Autodesk Fusion 360 part; units mm, degrees
(part 2 of 2)
  line L878 (-48.8114, -148.3999) -> (-48.8431, -148.4136)
  line L879 (-43.0004, -145.5999) -> (-42.9905, -145.5999)
  line L880 (-36.8003, -145.5886) -> (-36.8155, -145.5568)
  line L881 (-30.959, -145.5847) -> (-30.9633, -145.5625)
  line L882 (-48.8004, -145.5999) -> (-48.8004, -145.5886)
  line L883 (-36.8003, -148.4094) -> (-36.8003, -148.3999)
  line L884 (-48.8004, -148.3999) -> (-48.8114, -148.3999)
  line L885 (-36.8003, -148.3999) -> (-36.8116, -148.3999)
  line L886 (-30.9633, -145.5625) -> (-30.9866, -145.5568)
  line L887 (-42.9591, -148.4136) -> (-42.9905, -148.3999)
  line L888 (-24.812, -148.3999) -> (-24.843, -148.4136)
  line L889 (-36.8116, -148.3999) -> (-36.8434, -148.4136)
  line L890 (-36.8377, -148.4373) -> (-36.8155, -148.4411)
  line L891 (-42.9867, -148.4411) -> (-42.963, -148.4373)
  line L892 (-24.812, -145.5999) -> (-24.801, -145.5999)
  line L893 (-36.8155, -148.4411) -> (-36.8003, -148.4094)
  line L894 (-48.8004, -148.4094) -> (-48.8004, -148.3999)
  line L895 (-24.801, -145.5999) -> (-19, -145.5999)
  line L896 (-36.8434, -148.4136) -> (-36.8377, -148.4373)
  line L897 (-36.8003, -148.3999) -> (-36.8003, -145.5999)
  line L898 (-48.8004, -145.5999) -> (-43.0004, -145.5999)
  line L899 (-48.8431, -145.5847) -> (-48.8114, -145.5999)
  line L900 (-24.801, -148.3999) -> (-24.801, -145.5999)
  line L901 (-48.8114, -145.5999) -> (-48.8004, -145.5999)
  line L902 (-42.9905, -148.3999) -> (-43.0004, -148.3999)
  line L903 (-48.8004, -145.5886) -> (-48.8156, -145.5568)
  line L904 (-43.0004, -148.3999) -> (-43.0004, -148.4094)
  line L905 (-42.963, -148.4373) -> (-42.9591, -148.4136)
  line L906 (-42.9591, -145.5847) -> (-42.963, -145.5625)
  line L907 (-24.801, -148.4094) -> (-24.801, -148.3999)
  line L908 (-31.0003, -148.4094) -> (-30.9866, -148.4411)
  line L909 (-24.843, -148.4136) -> (-24.838, -148.4373)
  line L910 (-24.801, -145.5999) -> (-24.801, -145.5886)
  line L911 (-33.8998, -148.3999) -> (-36.8003, -148.3999)
  line L912 (-42.9867, -145.5568) -> (-43.0004, -145.5886)
  line L913 (-43.0004, -145.5999) -> (-43.0004, -148.3999)
  line L914 (-57.544, -159.1843) -> (-57.5123, -159.1995)
  line L915 (-24.838, -148.4373) -> (-24.816, -148.4411)
  line L916 (-21.9, -148.3999) -> (-24.801, -148.3999)
  line L917 (-36.8377, -145.5625) -> (-36.8434, -145.5847)
  line L918 (-24.801, -145.5886) -> (-24.816, -145.5568)
  line L919 (-94.5377, -195.1374) -> (-94.5155, -195.1416)
  line L920 (-94.5003, -192.289) -> (-94.5155, -192.2573)
  line L921 (-36.8003, -145.5999) -> (-31.0003, -145.5999)
  line L922 (-106.5003, -192.3001) -> (-100.7001, -192.3001)
  line L923 (-106.5113, -195.1002) -> (-106.543, -195.114)
  line L924 (-94.5003, -195.1002) -> (-94.5003, -192.3001)
  line L925 (-31.0003, -145.5999) -> (-30.9908, -145.5999)
  line L926 (-100.7001, -192.289) -> (-100.7001, -192.3001)
  line L927 (-100.6905, -195.1002) -> (-100.7001, -195.1002)
  line L928 (-100.7001, -195.1002) -> (-103.5996, -195.1002)
  line L929 (-100.7001, -192.3001) -> (-100.6905, -192.3001)
  line L930 (-119.5999, -200.0005) -> (-119.5999, -209.9996)
  line L931 (-106.5155, -195.1416) -> (-106.5003, -195.1099)
  line L932 (-100.6629, -195.1374) -> (-100.6588, -195.114)
  line L933 (-36.8116, -145.5999) -> (-36.8003, -145.5999)
  line L934 (-94.5113, -195.1002) -> (-94.543, -195.114)
  line L935 (-94.5003, -195.1099) -> (-94.5003, -195.1002)
  line L936 (-106.543, -192.2849) -> (-106.5113, -192.3001)
  line L937 (-106.5003, -195.1002) -> (-106.5003, -192.3001)
  line L938 (-106.5375, -195.1374) -> (-106.5155, -195.1416)
  line L939 (-100.6588, -195.114) -> (-100.6905, -195.1002)
  line L940 (-94.5003, -192.3001) -> (-94.5003, -192.289)
  line L941 (-100.7001, -195.1002) -> (-100.7001, -195.1099)
  line L942 (-119.5999, -209.9996) -> (-19.6, -209.9996)
  line L943 (-94.5113, -192.3001) -> (-94.5003, -192.3001)
  line L944 (-103.5996, -195.1002) -> (-106.5003, -195.1002)
  line L945 (-94.5155, -192.2573) -> (-94.5377, -192.2615)
  line L946 (-94.5003, -195.1002) -> (-94.5113, -195.1002)
  line L947 (-88.7003, -192.3001) -> (-88.6904, -192.3001)
  line L948 (-88.6904, -192.3001) -> (-88.6587, -192.2849)
  line L949 (-106.5003, -192.289) -> (-106.5155, -192.2573)
  line L950 (-94.5377, -192.2615) -> (-94.543, -192.2849)
  line L951 (-88.6587, -192.2849) -> (-88.6629, -192.2615)
  line L952 (-100.6905, -192.3001) -> (-100.6588, -192.2849)
  line L953 (-106.543, -195.114) -> (-106.5375, -195.1374)
  line L954 (-82.5154, -195.1416) -> (-82.5002, -195.1099)
  line L955 (-76.6865, -192.2573) -> (-76.7002, -192.289)
  line L956 (-63.6005, -198.3) -> (-63.5839, -198.3)
  line L957 (-106.5003, -192.3001) -> (-106.5003, -192.289)
  line L958 (-76.7002, -192.3001) -> (-76.7002, -195.1002)
  line L959 (-36.8434, -145.5847) -> (-36.8116, -145.5999)
  line L960 (-19.6, -200.0005) -> (-119.5999, -200.0005)
  line L961 (-100.7001, -192.3001) -> (-100.7001, -195.1002)
  line L962 (-94.543, -195.114) -> (-94.5377, -195.1374)
  line L963 (-94.5155, -195.1416) -> (-94.5003, -195.1099)
  line L964 (-106.5113, -192.3001) -> (-106.5003, -192.3001)
  line L965 (-24.838, -145.5625) -> (-24.843, -145.5847)
  line L966 (-100.7001, -195.1099) -> (-100.6864, -195.1416)
  line L967 (-106.5375, -192.2615) -> (-106.543, -192.2849)
  line L968 (-91.5994, -195.1002) -> (-94.5003, -195.1002)
  line L969 (-100.6864, -195.1416) -> (-100.6629, -195.1374)
  line L970 (-94.543, -192.2849) -> (-94.5113, -192.3001)
  line L971 (-94.5003, -192.3001) -> (-88.7003, -192.3001)
  line L972 (-106.5003, -195.1099) -> (-106.5003, -195.1002)
  line L973 (-76.6907, -192.3001) -> (-76.6589, -192.2849)
  line L974 (-100.6588, -192.2849) -> (-100.6629, -192.2615)
  line L975 (-24.816, -145.5568) -> (-24.838, -145.5625)
  line L976 (-106.5003, -195.1002) -> (-106.5113, -195.1002)
  line L977 (-100.6629, -192.2615) -> (-100.6864, -192.2573)
  line L978 (-106.5155, -192.2573) -> (-106.5375, -192.2615)
  line L979 (-100.6864, -192.2573) -> (-100.7001, -192.289)
  line L980 (-19.6, -209.9996) -> (-19.6, -200.0005)
  line L981 (-82.5002, -195.1099) -> (-82.5002, -195.1002)
  line L982 (-88.7003, -195.1002) -> (-91.5994, -195.1002)
  line L983 (-88.6629, -192.2615) -> (-88.6865, -192.2573)
  line L984 (-63.5, -198.1994) -> (-63.5, -189.1995)
  line L985 (-76.7002, -192.289) -> (-76.7002, -192.3001)
  line L986 (-63.5839, -189.1003) -> (-63.6005, -189.1003)
  line L987 (-63.6005, -189.1003) -> (-66.5, -189.1003)
  line L988 (-82.5376, -192.2615) -> (-82.5433, -192.2849)
  line L989 (-58.9992, -136.4097) -> (-58.9855, -136.4414)
  line L990 (-58.958, -124.4138) -> (-58.9897, -124.4)
  line L991 (-58.958, -136.4135) -> (-58.9897, -136.3998)
  line L992 (-17.416, -114.752) -> (-17.607, -114.989)
  line L993 (-58.9855, -136.4414) -> (-58.9622, -136.4372)
  line L994 (-58.9897, -124.4) -> (-58.9992, -124.4)
  line L995 (-61.9181, -124.4) -> (-61.9703, -124.429)
  line L996 (-18.597, -115.4) -> (-58.9001, -115.4)
  line L997 (-17.844, -115.181) -> (-17.897, -115.213)
  line L998 (-61.9181, -136.3998) -> (-61.9703, -136.4287)
  line L999 (-61.9993, -130.5006) -> (-61.9993, -130.5172)
  line L1000 (-58.9992, -130.5998) -> (-58.9992, -136.3998)
  line L1001 (-17.353, -114.646) -> (-17.384, -114.7)
  line L1002 (-17.148, -113.254) -> (-17.196, -113.812)
  line L1003 (-58.9622, -124.4371) -> (-58.958, -124.4138)
  line L1004 (-58.9622, -136.4372) -> (-58.958, -136.4135)
  line L1005 (-58.9992, -115.501) -> (-58.9992, -124.4)
  line L1006 (-58.9855, -130.5571) -> (-58.9992, -130.5888)
  line L1007 (-58.9622, -130.5627) -> (-58.9855, -130.5571)
  line L1008 (-17.95, -115.243) -> (-18.234, -115.352)
  line L1009 (-17.196, -114.089) -> (-17.245, -114.362)
  line L1010 (-58.9992, -142.5999) -> (-58.9897, -142.5999)
  line L1011 (-58.9992, -124.4) -> (-61.9001, -124.4)
  line L1012 (-61.9703, -130.5708) -> (-61.9181, -130.5998)
  line L1013 (-17.004, -112.524) -> (-17.148, -113.254)
  line L1014 (-58.9001, -115.4) -> (-58.9181, -115.4)
  line L1015 (-58.9181, -115.4) -> (-58.9703, -115.429)
  line L1016 (-58.9703, -115.429) -> (-58.9992, -115.483)
  line L1017 (-61.9001, -136.3998) -> (-61.9181, -136.3998)
  line L1018 (-12.735, -112.462) -> (-12.74, -112.485)
  line L1019 (-58.9992, -136.3998) -> (-58.9992, -136.4097)
  line L1020 (-61.9993, -124.5006) -> (-61.9993, -130.5006)
  line L1021 (-58.9992, -151.517) -> (-58.9703, -151.5706)
  line L1022 (-10.299, -115.301) -> (-12.697, -115.301)
  line L1023 (-58.958, -130.5846) -> (-58.9622, -130.5627)
  line L1024 (-18.234, -115.352) -> (-18.507, -115.4)
  line L1025 (-61.9001, -124.4) -> (-61.9181, -124.4)
  line L1026 (-61.9703, -142.5709) -> (-61.9181, -142.5999)
  line L1027 (-61.9993, -124.4826) -> (-61.9993, -124.5006)
  line L1028 (-10.29, -115.301) -> (-10.299, -115.301)
  line L1029 (-10.258, -115.315) -> (-10.29, -115.301)
  line L1030 (-10.286, -112.458) -> (-10.299, -112.49)
  line L1031 (-58.9992, -130.5998) -> (-58.9897, -130.5998)
  line L1032 (-18.507, -115.4) -> (-18.597, -115.4)
  line L1033 (-10.286, -115.342) -> (-10.262, -115.338)
  line L1034 (-12.708, -115.301) -> (-12.74, -115.315)
  line L1035 (-12.697, -112.5) -> (-11.498, -112.5)
  line L1036 (-12.735, -115.338) -> (-12.712, -115.342)
  line L1037 (-61.9181, -130.5998) -> (-61.9001, -130.5998)
  line L1038 (-12.697, -115.301) -> (-12.697, -112.5)
  line L1039 (-17.607, -114.989) -> (-17.844, -115.181)
  line L1040 (-58.9897, -130.5998) -> (-58.958, -130.5846)
  line L1041 (-58.9897, -142.5999) -> (-58.958, -142.5847)
  line L1042 (-61.9703, -124.429) -> (-61.9993, -124.4826)
  line L1043 (-17.384, -114.7) -> (-17.416, -114.752)
  line L1044 (-61.9993, -142.5169) -> (-61.9703, -142.5709)
  line L1045 (-58.9992, -124.4) -> (-58.9992, -124.4096)
  line L1046 (-58.9622, -142.5625) -> (-58.9855, -142.5572)
  line L1047 (-61.9001, -130.5998) -> (-58.9992, -130.5998)
  line L1048 (-17.196, -113.812) -> (-17.196, -114)
  line L1049 (-58.9992, -115.483) -> (-58.9992, -115.501)
  line L1050 (-58.9855, -124.4413) -> (-58.9622, -124.4371)
  line L1051 (-17.897, -115.213) -> (-17.95, -115.243)
  line L1052 (-58.9992, -124.4096) -> (-58.9855, -124.4413)
  line L1053 (-10.299, -112.5) -> (-10.29, -112.5)
  line L1054 (-58.9992, -142.5886) -> (-58.9992, -142.5999)
  line L1055 (-12.697, -115.31) -> (-12.697, -115.301)
  line L1056 (-12.74, -112.485) -> (-12.708, -112.5)
  line L1057 (-10.258, -112.485) -> (-10.262, -112.462)
  line L1058 (-10.262, -112.462) -> (-10.286, -112.458)
  line L1059 (-18.991, -145.5999) -> (-18.959, -145.5847)
  line L1060 (-10.299, -112.5) -> (-10.299, -115.301)
  line L1061 (-12.712, -115.342) -> (-12.697, -115.31)
  line L1062 (-58.9181, -151.5996) -> (-58.9001, -151.5996)
  line L1063 (-18.959, -145.5847) -> (-18.963, -145.5625)
  line L1064 (-58.9992, -142.5999) -> (-58.9992, -151.5004)
  line L1065 (-10.299, -115.31) -> (-10.286, -115.342)
  line L1066 (-58.9703, -151.5706) -> (-58.9181, -151.5996)
  line L1067 (-10.262, -115.338) -> (-10.258, -115.315)
  line L1068 (-11.498, -112.5) -> (-10.299, -112.5)
  line L1069 (-12.697, -112.5) -> (-12.697, -112.49)
  line L1070 (-10.29, -112.5) -> (-10.258, -112.485)
  line L1071 (-58.9855, -142.5572) -> (-58.9992, -142.5886)
  line L1072 (-58.9992, -151.5004) -> (-58.9992, -151.517)
  line L1073 (-58.958, -142.5847) -> (-58.9622, -142.5625)
  line L1074 (-10.299, -112.49) -> (-10.299, -112.5)
  line L1075 (-12.697, -112.49) -> (-12.712, -112.458)
  line L1076 (-12.697, -115.301) -> (-12.708, -115.301)
  line L1077 (-12.74, -115.315) -> (-12.735, -115.338)
  line L1078 (-10.299, -115.301) -> (-10.299, -115.31)
  line L1079 (-12.708, -112.5) -> (-12.697, -112.5)
  line L1080 (-12.712, -112.458) -> (-12.735, -112.462)
  line L1081 (-19, -145.5999) -> (-18.991, -145.5999)
  line L1082 (-8.829, -115.429) -> (-8.883, -115.4)
  line L1083 (-10.077, -116.53) -> (-10.168, -116.578)
  line L1084 (-13.862, -115.681) -> (-14.075, -115.328)
  line L1085 (-10.261, -116.625) -> (-10.55, -116.739)
  line L1086 (-8.837, -124.4371) -> (-8.815, -124.4413)
  line L1087 (-14.341, -113.416) -> (-14.316, -113.316)
  line L1088 (-8.883, -115.4) -> (-8.899, -115.4)
  line L1089 (-14.238, -114.948) -> (-14.272, -114.85)
  line L1090 (-8.899, -115.4) -> (-8.921, -115.4)
  line L1091 (-11.672, -116.896) -> (-11.774, -116.887)
  line L1092 (-61.9993, -130.5172) -> (-61.9703, -130.5708)
  line L1093 (-17.196, -114) -> (-17.196, -114.089)
  line L1094 (-9, -115.513) -> (-8.989, -115.546)
  line L1095 (-9.077, -112.401) -> (-8.921, -112.672)
  line L1096 (-8.649, -109.065) -> (-8.811, -108.971)
  line L1097 (-13.575, -111.971) -> (-13.499, -111.901)
  line L1098 (-5.8, -115.517) -> (-5.8, -115.501)
  line L1099 (-16.018, -110.53) -> (-16.341, -110.99)
  line L1100 (-9.137, -112.317) -> (-9.077, -112.401)
  line L1101 (-8.921, -112.672) -> (-8.759, -113.05)
  line L1102 (-5.829, -115.571) -> (-5.8, -115.517)
  line L1103 (-8.912, -115.6) -> (-8.899, -115.6)
  line L1104 (-8.811, -108.971) -> (-9.32, -108.735)
  line L1105 (-8.759, -113.05) -> (-8.651, -113.45)
  line L1106 (-16.764, -111.82) -> (-17.004, -112.524)
  line L1107 (-53.5284, -161.5504) -> (-53.5615, -161.6484)
  line L1108 (-58.3036, -162.7978) -> (-58.5819, -162.493)
  line L1109 (-58.958, -171.1142) -> (-58.9897, -171.1004)
  line L1110 (-55.1021, -161.9998) -> (-55.1021, -162.0093)
  line L1111 (-61.9181, -177.3001) -> (-61.9001, -177.3001)
  line L1112 (-61.9001, -171.1004) -> (-61.9181, -171.1004)
  line L1113 (-58.7622, -162.2383) -> (-58.8133, -162.1501)
  line L1114 (-57.9864, -163.061) -> (-58.3036, -162.7978)
  line L1115 (-58.9992, -162.1995) -> (-58.9992, -171.1004)
  line L1116 (-58.958, -177.285) -> (-58.9622, -177.2617)
  line L1117 (-53.9404, -162.3815) -> (-54.2039, -162.6997)
  line L1118 (-58.9992, -183.1002) -> (-58.9992, -183.11)
  line L1119 (-57.5402, -163.3241) -> (-57.6308, -163.2772)
  line L1120 (-61.9703, -177.2698) -> (-61.9181, -177.3001)
  line L1121 (-58.8133, -162.1501) -> (-58.819, -162.1416)
  line L1122 (-58.819, -162.1416) -> (-58.8807, -162.1003)
  line L1123 (-56.8508, -163.5474) -> (-57.2505, -163.4398)
  line L1124 (-55.9248, -163.5764) -> (-56.0267, -163.5873)
  line L1125 (-53.4596, -160.116) -> (-53.4155, -160.4247)
  line L1126 (-58.5819, -162.493) -> (-58.7622, -162.2383)
  line L1127 (-58.8807, -162.1003) -> (-58.9001, -162.1003)
  line L1128 (-58.9897, -177.3001) -> (-58.958, -177.285)
  line L1129 (-58.9622, -171.1375) -> (-58.958, -171.1142)
  line L1130 (-55.6175, -163.5171) -> (-55.9248, -163.5764)
  line L1131 (-58.9001, -162.1003) -> (-58.9181, -162.1003)
  line L1132 (-56.1301, -163.5968) -> (-56.4416, -163.5954)
  line L1133 (-53.4553, -161.2473) -> (-53.5284, -161.5504)
  line L1134 (-58.9855, -171.1417) -> (-58.9622, -171.1375)
  line L1135 (-58.9992, -171.1004) -> (-61.9001, -171.1004)
  line L1136 (-58.9992, -171.1099) -> (-58.9855, -171.1417)
  line L1137 (-53.5079, -159.9163) -> (-53.4832, -160.0168)
  line L1138 (-5.8, -114) -> (-5.8, -113.812)
  line L1139 (-12.244, -108.35) -> (-12.974, -108.495)
  line L1140 (-9, -115.488) -> (-9, -115.501)
  line L1141 (-8.986, -115.45) -> (-8.989, -115.453)
  line L1142 (-10.754, -108.35) -> (-11.312, -108.302)
  line L1143 (-11.312, -108.302) -> (-11.498, -108.302)
  line L1144 (-11.498, -108.302) -> (-11.686, -108.302)
  line L1145 (-8.651, -113.45) -> (-8.607, -113.759)
  line L1146 (-14.187, -108.971) -> (-14.347, -109.065)
  line L1147 (-8.955, -115.583) -> (-8.95, -115.586)
  line L1148 (-8.598, -113.964) -> (-8.613, -114.276)
  line L1149 (-14.968, -109.48) -> (-15.528, -109.97)
  line L1150 (-14.347, -109.065) -> (-14.508, -109.158)
  line L1151 (-13.679, -108.735) -> (-14.187, -108.971)
  line L1152 (-61.9703, -171.1293) -> (-61.9993, -171.1816)
  line L1153 (-53.5615, -161.6484) -> (-53.5961, -161.7447)
  line L1154 (-57.6308, -163.2772) -> (-57.7232, -163.2289)
  line L1155 (-61.9993, -171.1995) -> (-61.9993, -177.1996)
  line L1156 (-58.9855, -177.2574) -> (-58.9992, -177.2892)
  line L1157 (-58.9992, -177.2892) -> (-58.9992, -177.3001)
  line L1158 (-58.9897, -171.1004) -> (-58.9992, -171.1004)
  line L1159 (-58.9992, -177.3001) -> (-58.9992, -183.1002)
  line L1160 (-61.9993, -171.1816) -> (-61.9993, -171.1995)
  line L1161 (-61.9993, -177.2162) -> (-61.9703, -177.2698)
  line L1162 (-54.8541, -163.2109) -> (-55.2249, -163.3915)
  line L1163 (-56.4416, -163.5954) -> (-56.8508, -163.5474)
  line L1164 (-57.2505, -163.4398) -> (-57.5402, -163.3241)
  line L1165 (-53.4832, -160.0168) -> (-53.4596, -160.116)
  line L1166 (-58.9181, -162.1003) -> (-58.9703, -162.1293)
  line L1167 (-61.9993, -136.4827) -> (-61.9993, -136.5007)
  line L1168 (-61.9993, -136.5007) -> (-61.9993, -142.5004)
  line L1169 (-58.9992, -136.3998) -> (-61.9001, -136.3998)
  line L1170 (-58.9992, -130.5888) -> (-58.9992, -130.5998)
  line L1171 (-76.5157, -69.741) -> (-76.5005, -69.71)
  line L1172 (-82.6629, -69.737) -> (-82.659, -69.714)
  line L1173 (-94.6905, -69.7) -> (-94.7, -69.7)
  line L1174 (-94.7, -69.7) -> (-100.5003, -69.7)
  line L1175 (-63.6005, -79.701) -> (-66.5, -79.701)
  line L1176 (-63.5839, -79.701) -> (-63.6005, -79.701)
  line L1177 (-94.6174, -66.7) -> (-94.6711, -66.729)
  line L1178 (-94.7, -69.7) -> (-94.7, -69.71)
  line L1179 (-66.5152, -79.742) -> (-66.5, -79.71)
  line L1180 (-82.7003, -66.799) -> (-82.7003, -69.7)
  line L1181 (-66.5, -79.701) -> (-66.5, -69.799)
  line L1182 (-88.5377, -69.737) -> (-88.5154, -69.741)
  line L1183 (-63.5, -79.782) -> (-63.5303, -79.73)
  line L1184 (-76.5005, -69.7) -> (-76.5005, -66.799)
  line L1185 (-82.6174, -66.7) -> (-82.6713, -66.729)
  line L1186 (-66.5825, -69.7) -> (-66.5991, -69.7)
  line L1187 (-76.5115, -69.7) -> (-76.5432, -69.714)
  line L1188 (-82.6907, -69.7) -> (-82.7003, -69.7)
  line L1189 (-100.5155, -69.741) -> (-100.5003, -69.71)
  line L1190 (-116.7006, -91.71) -> (-116.6868, -91.742)
  line L1191 (-76.5376, -69.737) -> (-76.5157, -69.741)
  line L1192 (-82.659, -69.714) -> (-82.6907, -69.7)
  line L1193 (-88.5003, -69.7) -> (-88.5116, -69.7)
  line L1194 (-82.5997, -66.7) -> (-82.6174, -66.7)
  line L1195 (-94.7, -69.71) -> (-94.6862, -69.741)
  line L1196 (-94.6711, -66.729) -> (-94.7, -66.782)
  line L1197 (-76.5005, -69.7) -> (-76.5115, -69.7)
  line L1198 (-66.5, -79.71) -> (-66.5, -79.701)
  line L1199 (-94.663, -69.737) -> (-94.6587, -69.714)
  line L1200 (-94.6587, -69.714) -> (-94.6905, -69.7)
  line L1201 (-66.5, -79.701) -> (-66.5109, -79.701)
  line L1202 (-76.5997, -66.7) -> (-82.5997, -66.7)
  line L1203 (-82.7003, -66.782) -> (-82.7003, -66.799)
  line L1204 (-94.6862, -69.741) -> (-94.663, -69.737)
  line L1205 (-8.935, -115.36) -> (-8.986, -115.45)
  line L1206 (-5.994, -112.524) -> (-6.234, -111.82)
  line L1207 (-14.508, -109.158) -> (-14.968, -109.48)
  line L1208 (-61.9703, -136.4287) -> (-61.9993, -136.4827)
  line L1209 (-6.234, -111.82) -> (-6.471, -111.311)
  line L1210 (-6.657, -110.989) -> (-6.98, -110.53)
  line L1211 (-7.47, -109.97) -> (-8.028, -109.48)
  line L1212 (-8.947, -115.587) -> (-8.912, -115.6)
  line L1213 (-5.883, -115.6) -> (-5.829, -115.571)
  line L1214 (-5.85, -113.254) -> (-5.994, -112.524)
  line L1215 (-53.4059, -160.8381) -> (-53.4553, -161.2473)
  line L1216 (-61.9993, -177.1996) -> (-61.9993, -177.2162)
  line L1217 (-54.5098, -162.9795) -> (-54.5909, -163.043)
  line L1218 (-58.9622, -177.2617) -> (-58.9855, -177.2574)
  line L1219 (-58.8807, -159.372) -> (-58.7251, -159.1017)
  line L1220 (-61.9181, -162.3) -> (-61.9001, -162.3)
  line L1221 (-58.8161, -162.2535) -> (-58.8133, -162.2506)
  line L1222 (-59.1993, -160.5626) -> (-59.195, -160.4592)
  line L1223 (-61.9509, -159.9548) -> (-61.9993, -160.5128)
  line L1224 (-54.4297, -162.9149) -> (-54.5098, -162.9795)
  line L1225 (-61.9993, -160.7002) -> (-61.9993, -162.1995)
  line L1226 (-61.9181, -171.1004) -> (-61.9703, -171.1293)
  line L1227 (-58.9992, -177.3001) -> (-58.9897, -177.3001)
  line L1228 (-61.9001, -177.3001) -> (-58.9992, -177.3001)
  line L1229 (-54.2039, -162.6997) -> (-54.4297, -162.9149)
  line L1230 (-58.9992, -162.1815) -> (-58.9992, -162.1995)
  line L1231 (-53.4155, -160.4247) -> (-53.4059, -160.8381)
  line L1232 (-53.5961, -161.7447) -> (-53.7256, -162.0287)
  line L1233 (-57.7232, -163.2289) -> (-57.9864, -163.061)
  line L1234 (-54.5909, -163.043) -> (-54.8541, -163.2109)
  line L1235 (-58.9703, -162.1293) -> (-58.9992, -162.1815)
  line L1236 (-53.7256, -162.0287) -> (-53.9404, -162.3815)
  line L1237 (-55.2249, -163.3915) -> (-55.6175, -163.5171)
  line L1238 (-58.9992, -171.1004) -> (-58.9992, -171.1099)
  line L1239 (-56.0267, -163.5873) -> (-56.1301, -163.5968)
  line L1240 (-82.6713, -66.729) -> (-82.7003, -66.782)
  line L1241 (-66.5152, -85.858) -> (-66.537, -85.862)
  line L1242 (-66.5109, -91.7) -> (-66.5427, -91.714)
  line L1243 (-66.5427, -85.885) -> (-66.5109, -85.9)
  line L1244 (-66.5, -103.7) -> (-66.5109, -103.7)
  line L1245 (-66.537, -91.738) -> (-66.5152, -91.742)
  line L1246 (-66.5, -103.7) -> (-66.5, -97.9)
  line L1247 (-63.6005, -97.9) -> (-63.5839, -97.9)
  line L1248 (-63.6005, -85.9) -> (-63.5839, -85.9)
  line L1249 (-66.5, -91.7) -> (-66.5, -85.9)
  line L1250 (-66.5109, -85.9) -> (-66.5, -85.9)
  line L1251 (-63.5839, -91.7) -> (-63.6005, -91.7)
  line L1252 (-63.5839, -85.9) -> (-63.5303, -85.87)
  line L1253 (-66.537, -85.862) -> (-66.5427, -85.885)
  line L1254 (-66.5, -119.817) -> (-66.5, -119.8)
  line L1255 (-66.5427, -91.714) -> (-66.537, -91.738)
  line L1256 (-66.5152, -103.742) -> (-66.5, -103.71)
  line L1257 (-66.537, -97.862) -> (-66.5427, -97.885)
  line L1258 (-66.5109, -109.9) -> (-66.5, -109.9)
  line L1259 (-63.5303, -85.87) -> (-63.5, -85.816)
  line L1260 (-66.5109, -97.9) -> (-66.5, -97.9)
  line L1261 (-63.5839, -103.7) -> (-63.6005, -103.7)
  line L1262 (-63.5, -109.816) -> (-63.5, -109.8)
  line L1263 (-66.5, -109.9) -> (-66.5, -109.889)
  line L1264 (-66.5, -97.9) -> (-66.5, -97.889)
  line L1265 (-63.5, -97.8) -> (-63.5, -91.8)
  line L1266 (-66.537, -109.862) -> (-66.5427, -109.885)
  line L1267 (-66.5, -109.9) -> (-63.6005, -109.9)
  line L1268 (-63.5, -91.782) -> (-63.5303, -91.729)
  line L1269 (-66.5303, -69.729) -> (-66.5825, -69.7)
  line L1270 (-55.3529, -157.9594) -> (-54.9726, -158.1221)
  line L1271 (-54.9726, -158.1221) -> (-54.6213, -158.3369)
  line L1272 (-59.1206, -161.3839) -> (-59.1894, -160.9757)
  line L1273 (-56.5781, -157.812) -> (-56.1661, -157.8021)
  line L1274 (-58.6645, -159.0178) -> (-58.6052, -158.9335)
  line L1275 (-59.1495, -160.1505) -> (-59.0433, -159.7508)
  line L1276 (-59.2046, -160.6645) -> (-59.1993, -160.5626)
  line L1277 (-55.8546, -157.8324) -> (-55.7526, -157.8533)
  line L1278 (-61.8063, -159.2245) -> (-61.9509, -159.9548)
  line L1279 (-59.1894, -160.9757) -> (-59.2046, -160.6645)
  line L1280 (-56.1661, -157.8021) -> (-55.8546, -157.8324)
  line L1281 (-58.8655, -162.0605) -> (-58.9954, -161.7765)
  line L1282 (-55.7526, -157.8533) -> (-55.6521, -157.8727)
  line L1283 (-58.6052, -158.9335) -> (-58.4013, -158.6967)
  line L1284 (-59.195, -160.4592) -> (-59.1495, -160.1505)
  line L1285 (-58.0954, -158.4195) -> (-57.7536, -158.188)
  line L1286 (-61.5668, -158.5204) -> (-61.8063, -159.2245)
  line L1287 (-58.7996, -162.1995) -> (-58.7996, -162.1871)
  line L1288 (-58.7996, -162.1871) -> (-58.8119, -162.1526)
  line L1289 (-58.8546, -162.2877) -> (-58.8504, -162.2863)
  line L1290 (-58.8479, -162.2838) -> (-58.8161, -162.2535)
  line L1291 (-58.8504, -162.2863) -> (-58.8479, -162.2838)
  line L1292 (-58.9001, -162.3) -> (-58.8878, -162.3)
  line L1293 (-61.9703, -162.2697) -> (-61.9181, -162.3)
  line L1294 (-61.3297, -158.0117) -> (-61.5668, -158.5204)
  line L1295 (-57.38, -158.0074) -> (-57.2851, -157.969)
  line L1296 (-56.9859, -157.8808) -> (-56.5781, -157.812)
  line L1297 (-55.6521, -157.8727) -> (-55.3529, -157.9594)
  line L1298 (-61.1434, -157.6892) -> (-61.2359, -157.8504)
  line L1299 (-58.8119, -162.2464) -> (-58.7996, -162.2104)
  line L1300 (-57.2851, -157.969) -> (-56.9859, -157.8808)
  line L1301 (-59.7725, -156.1804) -> (-60.3306, -156.6707)
  line L1302 (-58.8878, -162.3) -> (-58.8546, -162.2877)
  line L1303 (-58.4013, -158.6967) -> (-58.0954, -158.4195)
  line L1304 (-58.8133, -162.1501) -> (-58.8655, -162.0605)
  line L1305 (-61.9993, -162.1995) -> (-61.9993, -162.2161)
  line L1306 (-58.8119, -162.1526) -> (-58.8133, -162.1501)
  line L1307 (-50.6042, -160.5128) -> (-50.6539, -159.9548)
  line L1308 (-51.4614, -157.6892) -> (-51.7839, -157.2288)
  line L1309 (-8.815, -177.2574) -> (-8.837, -177.2617)
  line L1310 (-5.8, -171.1995) -> (-5.8, -171.1816)
  line L1311 (-8.8, -162.1815) -> (-8.829, -162.1293)
  line L1312 (-8.8, -171.1004) -> (-8.8, -162.1995)
  line L1313 (-53.6155, -155.6717) -> (-54.1238, -155.4346)
  line L1314 (-55.5582, -155.0504) -> (-56.1163, -155.0021)
  line L1315 (-8.815, -171.1417) -> (-8.8, -171.1099)
  line L1316 (-8.8, -177.3001) -> (-5.899, -177.3001)
  line L1317 (-8.843, -171.1142) -> (-8.837, -171.1375)
  line L1318 (-8.811, -177.3001) -> (-8.8, -177.3001)
  line L1319 (-8.8, -171.1099) -> (-8.8, -171.1004)
  line L1320 (-5.899, -171.1004) -> (-8.8, -171.1004)
  line L1321 (-5.883, -177.3001) -> (-5.829, -177.2698)
  line L1322 (-51.7839, -157.2288) -> (-52.2746, -156.6707)
  line L1323 (-17.245, -114.362) -> (-17.353, -114.646)
  line L1324 (-58.9897, -136.3998) -> (-58.9992, -136.3998)
  line L1325 (-58.8133, -162.2506) -> (-58.8119, -162.2464)
  line L1326 (-60.821, -157.2288) -> (-61.1434, -157.6892)
  line L1327 (-8.811, -171.1004) -> (-8.843, -171.1142)
  line L1328 (-49.9043, -161.913) -> (-49.9579, -161.8813)
  line L1329 (-8.843, -177.285) -> (-8.811, -177.3001)
  line L1330 (-8.8, -171.1004) -> (-8.811, -171.1004)
  line L1331 (-8.8, -162.1995) -> (-8.8, -162.1815)
  line L1332 (-50.6042, -160.7002) -> (-50.6042, -160.5128)
  line L1333 (-50.4155, -161.4004) -> (-50.4472, -161.3465)
  line L1334 (-5.8, -177.1996) -> (-5.8, -171.1995)
  line L1335 (-5.8, -171.1816) -> (-5.829, -171.1293)
  line L1336 (-58.7251, -159.1017) -> (-58.6645, -159.0178)
  line L1337 (-57.4766, -158.0448) -> (-57.38, -158.0074)
  line L1338 (-61.9993, -160.5128) -> (-61.9993, -160.7002)
  line L1339 (-59.3122, -155.8579) -> (-59.7725, -156.1804)
  line L1340 (-6.471, -111.311) -> (-6.564, -111.151)
  line L1341 (-5.8, -115.501) -> (-5.8, -114)
  line L1342 (-15.528, -109.97) -> (-16.018, -110.53)
  line L1343 (-8.607, -113.759) -> (-8.602, -113.862)
  line L1344 (-10.024, -108.495) -> (-10.754, -108.35)
  line L1345 (-119.7005, -79.8) -> (-119.7005, -85.8)
  line L1346 (-116.7006, -79.701) -> (-116.7006, -79.71)
  line L1347 (-106.6588, -69.714) -> (-106.6905, -69.7)
  line L1348 (-116.6592, -85.885) -> (-116.6633, -85.862)
  line L1349 (-119.7005, -85.816) -> (-119.6716, -85.87)
  line L1350 (-116.6868, -85.858) -> (-116.7006, -85.889)
  line L1351 (-116.7006, -85.889) -> (-116.7006, -85.9)
  line L1352 (-116.6633, -85.862) -> (-116.6868, -85.858)
  line L1353 (-119.5999, -85.9) -> (-116.7006, -85.9)
  line L1354 (-119.6716, -103.729) -> (-119.7005, -103.782)
  line L1355 (-116.6592, -109.885) -> (-116.6633, -109.862)
  line L1356 (-116.6633, -109.862) -> (-116.6868, -109.857)
  line L1357 (-116.6179, -69.7) -> (-116.6716, -69.729)
  line L1358 (-100.5293, -66.729) -> (-100.583, -66.7)
  line L1359 (-106.7001, -66.782) -> (-106.7001, -66.799)
  line L1360 (-119.6179, -79.701) -> (-119.6716, -79.73)
  line L1361 (-106.6864, -69.741) -> (-106.6629, -69.737)
  line L1362 (-100.5114, -69.7) -> (-100.5431, -69.714)
  line L1363 (-106.6905, -69.7) -> (-106.7001, -69.7)
  line L1364 (-3.6005, -61.696) -> (-6.5, -61.696)
  line L1365 (-3.5, -61.795) -> (-3.5, -61.777)
  line L1366 (-116.6909, -109.9) -> (-116.6592, -109.885)
  line L1367 (-116.7006, -91.7) -> (-116.7006, -91.71)
  line L1368 (-119.7005, -85.8) -> (-119.7005, -85.816)
  line L1369 (-116.6592, -79.714) -> (-116.6909, -79.701)
  line L1370 (-119.7005, -79.782) -> (-119.7005, -79.8)
  line L1371 (-116.6716, -119.87) -> (-116.6179, -119.901)
  line L1372 (-119.7005, -97.816) -> (-119.6716, -97.87)
  line L1373 (-6.5, -61.696) -> (-6.5109, -61.696)
  line L1374 (-116.7006, -109.889) -> (-116.7006, -109.9)
  line L1375 (-100.5003, -69.71) -> (-100.5003, -69.7)
  line L1376 (-116.6592, -97.885) -> (-116.6633, -97.862)
  line L1377 (-3.5303, -105.17) -> (-3.5, -105.117)
  line L1378 (-119.5999, -79.701) -> (-119.6179, -79.701)
  line L1379 (-116.7006, -69.782) -> (-116.7006, -69.799)
  line L1380 (-3.5839, -61.696) -> (-3.6005, -61.696)
  line L1381 (-116.7006, -79.701) -> (-119.5999, -79.701)
  line L1382 (-119.5999, -109.9) -> (-116.7006, -109.9)
  line L1383 (-119.7005, -97.8) -> (-119.7005, -97.816)
  line L1384 (-116.6179, -119.901) -> (-116.5999, -119.901)
  line L1385 (-6.537, -61.733) -> (-6.5152, -61.737)
  line L1386 (-6.5152, -56.055) -> (-6.537, -56.058)
  line L1387 (-6.5109, -61.696) -> (-6.5427, -61.71)
  line L1388 (-116.6909, -103.7) -> (-116.7006, -103.7)
  line L1389 (-116.6909, -97.9) -> (-116.6592, -97.885)
  line L1390 (-116.7006, -97.9) -> (-116.6909, -97.9)
  line L1391 (-116.6868, -91.742) -> (-116.6633, -91.738)
  line L1392 (-106.7001, -66.799) -> (-106.7001, -69.7)
  line L1393 (-116.6633, -91.738) -> (-116.6592, -91.714)
  line L1394 (-116.6633, -79.738) -> (-116.6592, -79.714)
  line L1395 (-116.6868, -79.742) -> (-116.6633, -79.738)
  line L1396 (-119.6179, -85.9) -> (-119.5999, -85.9)
  line L1397 (-116.7006, -85.9) -> (-116.7006, -91.7)
  line L1398 (-106.6629, -69.737) -> (-106.6588, -69.714)
  line L1399 (-116.6592, -91.714) -> (-116.6909, -91.7)
  line L1400 (-116.6909, -91.7) -> (-116.7006, -91.7)
  line L1401 (-116.7006, -91.7) -> (-119.5999, -91.7)
  line L1402 (-119.5999, -91.7) -> (-119.6179, -91.7)
  line L1403 (-100.5431, -69.714) -> (-100.5376, -69.737)
  line L1404 (-119.6716, -85.87) -> (-119.6179, -85.9)
  line L1405 (-116.7006, -69.799) -> (-116.7006, -79.701)
  line L1406 (-106.7001, -69.7) -> (-116.5999, -69.7)
  line L1407 (-116.5999, -69.7) -> (-116.6179, -69.7)
  line L1408 (-116.6909, -85.9) -> (-116.6592, -85.885)
  line L1409 (-106.7001, -69.71) -> (-106.6864, -69.741)
  line L1410 (-100.5376, -69.737) -> (-100.5155, -69.741)
  line L1411 (-116.6716, -69.729) -> (-116.7006, -69.782)
  line L1412 (-116.6909, -79.701) -> (-116.7006, -79.701)
  line L1413 (-119.6716, -79.73) -> (-119.7005, -79.782)
  line L1414 (-106.6712, -66.729) -> (-106.7001, -66.782)
  line L1415 (-100.583, -66.7) -> (-100.5996, -66.7)
  line L1416 (-100.5003, -69.7) -> (-100.5003, -66.799)
  line L1417 (-106.7001, -69.7) -> (-106.7001, -69.71)
  line L1418 (-106.5995, -66.7) -> (-106.6174, -66.7)
  line L1419 (-100.5003, -66.782) -> (-100.5293, -66.729)
  line L1420 (-116.7006, -79.71) -> (-116.6868, -79.742)
  line L1421 (-116.7006, -85.9) -> (-116.6909, -85.9)
  line L1422 (-119.6716, -91.729) -> (-119.7005, -91.782)
  line L1423 (-100.5996, -66.7) -> (-106.5995, -66.7)
  line L1424 (-100.5003, -66.799) -> (-100.5003, -66.782)
  line L1425 (-100.5003, -69.7) -> (-100.5114, -69.7)
  line L1426 (-106.6174, -66.7) -> (-106.6712, -66.729)
  line L1427 (-119.6179, -91.7) -> (-119.6716, -91.729)
  line L1428 (-119.7005, -91.782) -> (-119.7005, -91.8)
  line L1429 (-19, -195.1002) -> (-21.9, -195.1002)
  line L1430 (-24.801, -192.3001) -> (-24.801, -192.289)
  line L1431 (-18.991, -192.3001) -> (-18.959, -192.2849)
  line L1432 (-8.8, -189.289) -> (-8.815, -189.2574)
  line L1433 (-5.899, -189.3001) -> (-5.883, -189.3001)
  line L1434 (-8.899, -198.3) -> (-8.883, -198.3)
  line L1435 (-18.963, -192.2615) -> (-18.986, -192.2573)
  line L1436 (-24.843, -195.114) -> (-24.838, -195.1374)
  line L1437 (-24.838, -195.1374) -> (-24.816, -195.1416)
  line L1438 (-18.959, -195.114) -> (-18.991, -195.1002)
  line L1439 (-30.9908, -195.1002) -> (-31.0003, -195.1002)
  line L1440 (-31.0003, -195.1002) -> (-33.8998, -195.1002)
  line L1441 (-8.843, -189.2849) -> (-8.811, -189.3001)
  line L1442 (-5.829, -189.2697) -> (-5.8, -189.216)
  line L1443 (-8.843, -183.1139) -> (-8.837, -183.1375)
  line L1444 (-8.8, -183.1002) -> (-8.8, -177.3001)
  line L1445 (-8.829, -198.2697) -> (-8.8, -198.216)
  line L1446 (-8.837, -189.2615) -> (-8.843, -189.2849)
  line L1447 (-5.899, -183.1002) -> (-8.8, -183.1002)
  line L1448 (-8.8, -183.11) -> (-8.8, -183.1002)
  line L1449 (-8.837, -183.1375) -> (-8.815, -183.1418)
  line L1450 (-19, -195.1002) -> (-19, -195.1099)
  line L1451 (-5.8, -189.1995) -> (-5.8, -183.1996)
  line L1452 (-8.8, -177.3001) -> (-8.8, -177.2892)
  line L1453 (-19, -192.289) -> (-19, -192.3001)
  line L1454 (-48.8431, -195.114) -> (-48.8378, -195.1374)
  line L1455 (-48.8004, -192.3001) -> (-43.0004, -192.3001)
  line L1456 (-36.8116, -195.1002) -> (-36.8434, -195.114)
  line L1457 (-36.8003, -192.289) -> (-36.8155, -192.2573)
  line L1458 (-42.9905, -195.1002) -> (-43.0004, -195.1002)
  line L1459 (-42.963, -195.1374) -> (-42.9591, -195.114)
  line L1460 (-36.8003, -195.1002) -> (-36.8116, -195.1002)
  line L1461 (-36.8155, -192.2573) -> (-36.8377, -192.2615)
  line L1462 (-36.8377, -195.1374) -> (-36.8155, -195.1416)
  line L1463 (-36.8155, -195.1416) -> (-36.8003, -195.1099)
  line L1464 (-48.8378, -195.1374) -> (-48.8156, -195.1416)
  line L1465 (-59.6716, -61.725) -> (-59.7005, -61.777)
  line L1466 (-33.8998, -195.1002) -> (-36.8003, -195.1002)
  line L1467 (-48.8004, -195.1002) -> (-48.8114, -195.1002)
  line L1468 (-36.8434, -192.2849) -> (-36.8116, -192.3001)
  line L1469 (-48.8378, -192.2615) -> (-48.8431, -192.2849)
  line L1470 (-59.7005, -61.777) -> (-59.7005, -61.795)
  line L1471 (-43.0004, -192.3001) -> (-43.0004, -195.1002)
  line L1472 (-48.8114, -195.1002) -> (-48.8431, -195.114)
  line L1473 (-59.6179, -105.199) -> (-59.5999, -105.199)
  line L1474 (-48.8004, -192.3001) -> (-48.8004, -192.289)
  line L1475 (-30.959, -192.2849) -> (-30.9633, -192.2615)
  line L1476 (-30.9633, -192.2615) -> (-30.9866, -192.2573)
  line L1477 (-30.9866, -192.2573) -> (-31.0003, -192.289)
  line L1478 (-31.0003, -192.3001) -> (-31.0003, -195.1002)
  line L1479 (-6.537, -56.058) -> (-6.5427, -56.082)
  line L1480 (-6.5109, -53.298) -> (-6.5427, -53.312)
  line L1481 (-56.7006, -52.082) -> (-56.7006, -52.1)
  line L1482 (-116.7006, -109.9) -> (-116.6909, -109.9)
  line L1483 (-3.5, -105.1) -> (-3.5, -102.1)
  line L1484 (-119.7005, -103.8) -> (-119.7005, -109.8)
  line L1485 (-116.6633, -103.738) -> (-116.6592, -103.714)
  line L1486 (-119.7005, -91.8) -> (-119.7005, -97.8)
  line L1487 (-116.7006, -119.8) -> (-116.7006, -119.817)
  line L1488 (-119.6179, -97.9) -> (-119.5999, -97.9)
  line L1489 (-119.6716, -109.87) -> (-119.6179, -109.9)
  line L1490 (-116.6868, -103.742) -> (-116.6633, -103.738)
  line L1491 (-116.7006, -103.7) -> (-119.5999, -103.7)
  line L1492 (-119.7005, -103.782) -> (-119.7005, -103.8)
  line L1493 (-116.7006, -103.71) -> (-116.6868, -103.742)
  line L1494 (-119.6179, -109.9) -> (-119.5999, -109.9)
  line L1495 (-116.6868, -109.857) -> (-116.7006, -109.889)
  line L1496 (-6.5991, -105.199) -> (-3.6005, -105.199)
  line L1497 (-3.6005, -105.199) -> (-3.5839, -105.199)
  line L1498 (-3.5303, -61.725) -> (-3.5839, -61.696)
  line L1499 (-6.5427, -61.71) -> (-6.537, -61.733)
  line L1500 (-116.7006, -109.9) -> (-116.7006, -119.8)
  line L1501 (-116.7006, -97.9) -> (-116.7006, -103.7)
  line L1502 (-116.6592, -103.714) -> (-116.6909, -103.7)
  line L1503 (-119.7005, -109.8) -> (-119.7005, -109.816)
  line L1504 (-116.7006, -97.889) -> (-116.7006, -97.9)
  line L1505 (-3.5, -102.1) -> (-3.5, -61.795)
  line L1506 (-119.7005, -109.816) -> (-119.6716, -109.87)
  line L1507 (-6.5, -61.706) -> (-6.5, -61.696)
  line L1508 (-116.6868, -97.858) -> (-116.7006, -97.889)
  line L1509 (-6.5, -61.696) -> (-6.5, -56.097)
  line L1510 (-6.5152, -61.737) -> (-6.5, -61.706)
  line L1511 (-116.7006, -103.7) -> (-116.7006, -103.71)
  line L1512 (-119.6716, -97.87) -> (-119.6179, -97.9)
  line L1513 (-6.5, -56.097) -> (-6.5, -56.086)
  line L1514 (-119.5999, -103.7) -> (-119.6179, -103.7)
  line L1515 (-119.6179, -103.7) -> (-119.6716, -103.729)
  line L1516 (-119.5999, -97.9) -> (-116.7006, -97.9)
  line L1517 (-116.7006, -119.817) -> (-116.6716, -119.87)
  line L1518 (-3.5, -61.777) -> (-3.5303, -61.725)
  line L1519 (-6.5, -56.086) -> (-6.5152, -56.055)
  line L1520 (-3.5839, -105.199) -> (-3.5303, -105.17)
  line L1521 (-3.5, -105.117) -> (-3.5, -105.1)
  line L1522 (-116.6633, -97.862) -> (-116.6868, -97.858)
  line L1523 (-56.7006, -61.696) -> (-56.7006, -61.706)
  line L1524 (-56.6868, -56.055) -> (-56.7006, -56.086)
  line L1525 (-56.7006, -56.086) -> (-56.7006, -56.097)
  line L1526 (-56.7006, -61.706) -> (-56.6868, -61.737)
  line L1527 (-56.6868, -61.737) -> (-56.6633, -61.733)
  line L1528 (-56.6592, -61.71) -> (-56.6909, -61.696)
  line L1529 (-94.7, -66.799) -> (-94.7, -69.7)
  line L1530 (-76.5831, -66.7) -> (-76.5997, -66.7)
  line L1531 (-76.5005, -66.799) -> (-76.5005, -66.782)
  line L1532 (-82.7003, -69.71) -> (-82.6865, -69.741)
  line L1533 (-88.5003, -69.7) -> (-88.5003, -66.799)
  line L1534 (-66.5427, -79.714) -> (-66.537, -79.738)
  line L1535 (-82.7003, -69.7) -> (-88.5003, -69.7)
  line L1536 (-82.6865, -69.741) -> (-82.6629, -69.737)
  line L1537 (-88.5292, -66.729) -> (-88.5832, -66.7)
  line L1538 (-76.5005, -66.782) -> (-76.5295, -66.729)
  line L1539 (-88.5003, -66.799) -> (-88.5003, -66.782)
  line L1540 (-66.5, -69.799) -> (-66.5, -69.782)
  line L1541 (-76.5005, -69.71) -> (-76.5005, -69.7)
  line L1542 (-63.5303, -79.73) -> (-63.5839, -79.701)
  line L1543 (-66.5, -69.782) -> (-66.5303, -69.729)
  line L1544 (-94.5995, -66.7) -> (-94.6174, -66.7)
  line L1545 (-88.5003, -66.782) -> (-88.5292, -66.729)
  line L1546 (-88.5832, -66.7) -> (-88.5998, -66.7)
  line L1547 (-76.5295, -66.729) -> (-76.5831, -66.7)
  line L1548 (-88.5998, -66.7) -> (-94.5995, -66.7)
  line L1549 (-94.7, -66.782) -> (-94.7, -66.799)
  line L1550 (-76.5432, -69.714) -> (-76.5376, -69.737)
  line L1551 (-66.5109, -79.701) -> (-66.5427, -79.714)
  line L1552 (-66.5991, -69.7) -> (-76.5005, -69.7)
  line L1553 (-88.5154, -69.741) -> (-88.5003, -69.71)
  line L1554 (-82.7003, -69.7) -> (-82.7003, -69.71)
  line L1555 (-66.537, -79.738) -> (-66.5152, -79.742)
  line L1556 (-88.5003, -69.71) -> (-88.5003, -69.7)
  line L1557 (-88.543, -69.714) -> (-88.5377, -69.737)
  line L1558 (-88.5116, -69.7) -> (-88.543, -69.714)
  line L1559 (-6.5991, -105.199) -> (-26.5995, -105.199)
  line L1560 (-36.5995, -105.199) -> (-56.5999, -105.199)
  line L1561 (-26.5995, -105.199) -> (-26.5995, -111.199)
  line L1562 (-36.5995, -105.199) -> (-36.5995, -111.199)
  circle A0 centre (-31.5995, -108.199) radius 2.5
  line L1563 (-26.5995, -111.199) -> (-36.5995, -111.199)
  line L1564 (-91.5995, -125.4) -> (-89.0995, -125.4)
  line L1565 (-89.0995, -125.4) -> (-89.0995, -128.4)
  line L1566 (-89.0995, -128.4) -> (-91.5995, -128.4)
  line L1567 (-91.5995, -125.4) -> (-94.0995, -125.4)
  line L1568 (-94.0995, -125.4) -> (-94.0995, -128.4)
  line L1569 (-94.0995, -128.4) -> (-91.5995, -128.4)
  line L1570 (-65.6396, -58.7128) -> (-65.6396, -61.7128)
  line L1571 (-70.6396, -61.7128) -> (-70.6396, -58.7128)
  line L1572 (-70.6396, -58.7128) -> (-65.6396, -58.7128)
  line L1573 (-70.6396, -67.7128) -> (-73.1396, -67.7128)
  line L1574 (-73.1396, -67.7128) -> (-73.1396, -61.7128)
  line L1575 (-73.1396, -61.7128) -> (-70.6396, -61.7128)
  line L1576 (-65.6396, -67.7128) -> (-63.1396, -67.7128)
  line L1577 (-63.1396, -67.7128) -> (-63.1396, -61.7128)
  line L1578 (-63.1396, -61.7128) -> (-65.6396, -61.7128)
  line L1579 (-70.6396, -67.7128) -> (-65.6396, -67.7128)
  circle A1 centre (-68.1396, -64.7128) radius 2.5
  point P0 (-31.5995, -105.199)
  dimension "d11" = 5
  dimension "d12" = 5
  dimension "d15" = 6
  dimension "d16" = 6
  dimension "d17" = 3
  dimension "d18" = 5
  dimension "d20" = 2.5
  dimension "d21" = 3
  dimension "d22" = 3
  dimension "d23" = 3
  dimension "d24" = 5
  dimension "d25" = 6
  dimension "d26" = 2.5
  dimension "d27" = 6
  dimension "d28" = 2.5
  dimension "d30" = 5
  constraint parallel L562 L1560
  constraint perpendicular L1559 L1561
  constraint perpendicular L1560 L1562
  constraint perpendicular L1562 L1563
  constraint horizontal L1564
  constraint vertical L1565
  constraint horizontal L1566
  constraint horizontal L1567
  constraint vertical L1568
  constraint horizontal L1569
  measures "d11" distance of P0 L1559.end
  measures "d12" distance of P0 L1560.start
  measures "d15" distance of L1559.end L1561.end
  measures "d16" distance of L1560.start L1562.end
  measures "d17" distance of P0 A0.centre
  measures "d18" diameter of A0
  measures "d20" distance of L1564.start L1564.end
  measures "d21" distance of L1564.start L1566.end
  measures "d22" distance of L1564.start L1566.end
  measures "d23" distance of L1570.start L1570.end
  measures "d24" distance of L1570.start L1571.end
  measures "d25" distance of L1571.start L1573.start
  measures "d26" distance of L1571.start L1574.end
  measures "d27" distance of L1570.end L1576.start
  measures "d28" distance of L1570.end L1577.end
  measures "d30" diameter of A1
